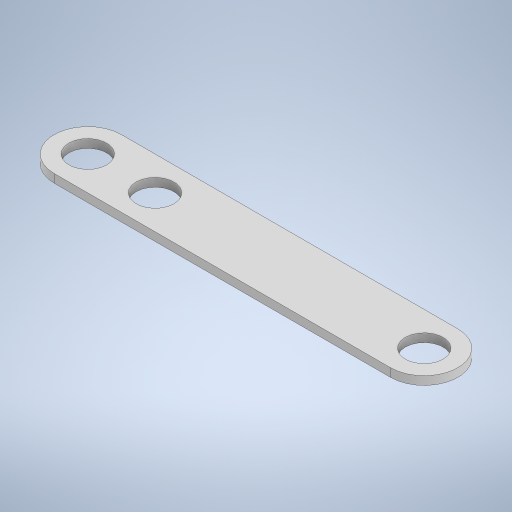
# Autodesk Inventor part: 4-bar intake block
Saved by Autodesk Inventor 2023 (Build 270158030, 158C)
## iProperties
Created: 2022-07-18
Part Number: 4-bar intake block
Material: Generic
Document SubType Name: Modeling
Designer: kt1040502
Density: 1 g/cm^3
Appearance: Default
Author: kt1040502
Autodesk Inventor part; units mm, degrees
ref_plane "YZ Plane" through (0, 0, 0) normal (1, 0, 0) x (0, 1, 0)
ref_plane "XZ Plane" through (0, 0, 0) normal (0, 1, 0) x (-1, 0, 0)
ref_plane "XY Plane" through (0, 0, 0) normal (0, 0, 1) x (1, 0, 0)
sketch "Sketch1" plane through (0, 0, 0) normal (0, 1, 0) x (-1, 0, 0)
  line L0 (0, 0) -> (-203.2, 0)
  line L1 (0, 25.4) -> (-76.2, 25.4) construction
  line L2 (-203.2, 25.4) -> (-127, 25.4) construction
  line L3 (-127, 25.4) -> (-330.2, 25.4)
  line L4 (0, 0) -> (-203.2, 0)
  line L5 (-203.2, 50.8) -> (0, 50.8)
  line L6 (-203.2, 0) -> (-330.2, 0)
  line L7 (-203.2, 50.8) -> (-330.2, 50.8)
  arc A0 (-330.2, 50.8) -> (-330.2, 0) centre (-330.2, 25.4) ccw
  arc A1 (0, 0) -> (0, 50.8) centre (0, 25.4) ccw
  arc A2 (-76.2, 0) -> (-76.2, 50.8) centre (-76.2, 25.4) ccw
  circle A3 centre (-330.2, 25.4) radius 14.2875
  circle A4 centre (-127, 25.4) radius 14.2875
  circle A5 centre (-76.2, 25.4) radius 14.2875
  point P0 (-331.4575, 38.0376)
  point P1 (-331.4575, 12.7624)
  point P2 (-76.2, 0)
  dimension "d2" = 76.2
  dimension "d3" = 76.2
  dimension "d8" = 203.2
  dimension "d12" = 50.8
  dimension "d17" = 28.575
  dimension "d18" = 28.575
  dimension "d19" = 28.575
  constraints: 16 end point, 7 horizontal, 6 centre point, 6 point on circle, 6 tangent, 3 coincident, 2 point on line, 1 parallel
  measures "d2" distance of L1.start L1.end
  measures "d3" distance of L2.start L2.end
  measures "d8" distance of L3.start L3.end
  measures "d12" distance of L4.end L5.start
  measures "d17" diameter of A3
  measures "d18" diameter of A4
  measures "d19" diameter of A5
extrude "Extrusion1" add sketch "Sketch1" along normal blind 6.35 contours L0 L6 A0 L7 L5 A2
body "Solid1"
